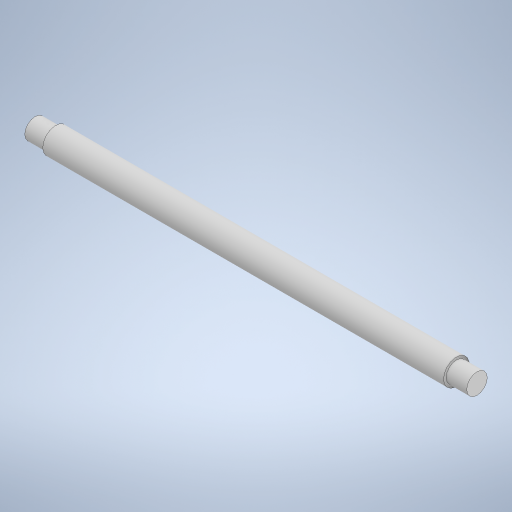
# Autodesk Inventor part: Manivelle
Saved by Autodesk Inventor 2023.2 (Build 272271030, 271C)
## iProperties
Created: 2023-03-02
Part Number: Manivelle
Material: Generic
Document SubType Name: Modeling
Designer: Luis Valente
Density: 1 g/cm^3
Appearance: Default
Author: Luis Valente
Autodesk Inventor part; units mm, degrees
ref_plane "YZ Plane" through (0, 0, 0) normal (1, 0, 0) x (0, 1, 0)
ref_plane "XZ Plane" through (0, 0, 0) normal (0, 1, 0) x (-1, 0, 0)
sketch "Sketch3" plane through (0, 0, 0) normal (0, 0, 1) x (1, 0, 0)
  line L0 (0, 0) -> (172, 0)
  line L1 (172, 0) -> (172, 4)
  line L2 (172, 4) -> (0, 4)
  line L3 (0, 4) -> (0, 0)
  dimension "d6" = 172
  dimension "d7" = 4
  constraints: 8 end point, 2 parallel, 1 horizontal, 1 perpendicular
  measures "d6" distance of L2.end L1.end
  measures "d7" distance of L1.end L0.end
revolve "Revolution1" add sketch "Sketch3" angle 360 about axis through (0, 0, 0) along (1, 0, 0)
ref_plane "Work Plane2" through (86, 0, 0) normal (-1, 0, 0) x (0, 0, 1)
sketch "Sketch6" plane through (86, 0, 0) normal (-1, 0, 0) x (0, 0, 1)
  circle A0 centre (0, 0) radius 5
  dimension "d12" = 10
  constraints: 1 centre point, 1 coincident
  measures "d12" diameter of A0
extrude "Extrusion2" add sketch "Sketch6" along normal blind 78 and the other way blind 78
body "Solid2"
